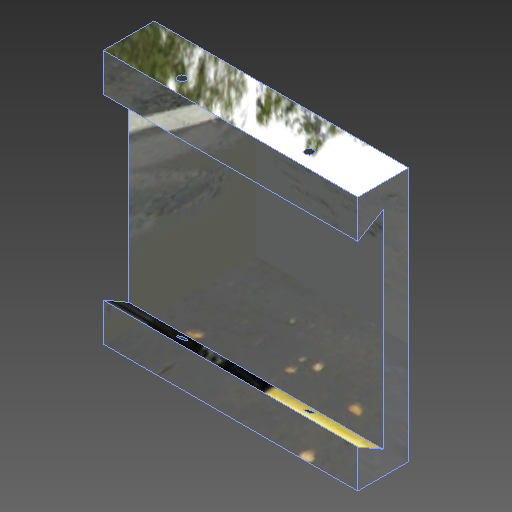
# Autodesk Inventor part: 3d_LM-Welding_Tooling - Fixed base
Saved by Autodesk Inventor 2018.3 (Build 223284000, 284)
## iProperties
Created: 2026-01-13
Part Number: 3d_LM-Welding_Tooling - Fixed base
Material: Aluminium 6061-T6
Document SubType Name: Modeling
Designer: aca6
Density: 2.7 g/cm^3
Appearance: N/A - Machined Aluminium
Manufacturer-1: {"Name": "Hanstar Technologies Co., Ltd", "PartNumber": "3d_Welding_Tooling - Fixed base", "Link": ""}
Manufacturer-2: {"Name": "SHENZHEN JINYIHE PROTOTYPE TECHNOLOGIES CO., LTD", "PartNumber": "3d_Welding_Tooling - Fixed base", "Link": ""}
Manufacturer-3: {"Name": "Shenzhen city Xavier Precision Co., Ltd.", "PartNumber": "3d_Welding_Tooling - Fixed base", "Link": ""}
Manufacturer-4: {"Name": "", "PartNumber": "", "Link": ""}
Manufacturer-5: {"Name": "", "PartNumber": "", "Link": ""}
Provider-1: {"Name": "", "PartNumber": "", "Link": ""}
Provider-2: {"Name": "", "PartNumber": "", "Link": ""}
Provider-3: {"Name": "", "PartNumber": "", "Link": ""}
Provider-4: {"Name": "", "PartNumber": "", "Link": ""}
Provider-5: {"Name": "", "PartNumber": "", "Link": ""}
Author: aca6
Comments: DIN-ISO-2768-fH
Autodesk Inventor part; units mm, degrees
ref_plane "YZ Plane" through (0, 0, 0) normal (1, 0, 0) x (0, 1, 0)
ref_plane "XZ Plane" through (0, 0, 0) normal (0, 1, 0) x (-1, 0, 0)
ref_plane "XY Plane" through (0, 0, 0) normal (0, 0, 1) x (1, 0, 0)
sketch "Sketch1" plane through (0, 0, 0) normal (0, 0, 1) x (1, 0, 0)
  line L0 (-50, 50) -> (50, 50)
  line L1 (50, 50) -> (50, -50)
  line L2 (50, -50) -> (-50, -50)
  line L3 (-50, -50) -> (-50, 50)
  line L4 (0, 0) -> (0, 7.629) construction
  line L5 (0, 0) -> (6.8797, 0) construction
  dimension "d0" = 100
  dimension "d1" = 100
  constraints: 12 end point, 3 horizontal, 2 parallel, 2 vertical, 1 perpendicular, 4 other
  measures "d0" distance between parallel lines of L2 L0
  measures "d1" distance between parallel lines of L1 L3
extrude "Extrusion1" add sketch "Sketch1" along normal blind 20
sketch "Sketch2" plane through (50, -50, 0) normal (1, 0, 0) x (0, 0, -1)
  line L0 (-20, 100) -> (-20, 0) projected
  line L1 (-20, 15) -> (-10, 9.2265)
  line L2 (-10, 9.2265) -> (-10, 90.7735)
  line L3 (-10, 90.7735) -> (-20, 85)
  line L4 (0, 0) -> (-20, 0) projected
  line L5 (0, 100) -> (-20, 100) projected
  point P0 (0, 50)
  dimension "d4" = 60
  dimension "d5" = 60
  dimension "d6" = 10
  dimension "d7" = 15
  dimension "d8" = 15
  constraints: 6 end point, 2 point on line, 1 parallel
  measures "d4" angle of L2 L1
  measures "d5" angle of L2 L3
  measures "d6" distance between parallel lines of L0 L2
  measures "d7" distance from line of L4 L1.start
  measures "d8" distance from line of L5 L3.end
extrude "Extrusion2" cut sketch "Sketch2" against normal blind 118.25
sketch "Sketch3" plane through (-50, -50, 0) normal (0, -1, 0) x (1, 0, 0)
  line L0 (100, 10) -> (0, 10) projected
  line L1 (0, 0) -> (0, 20) projected
  line L2 (0, 20) -> (100, 20) projected
  line L3 (100, 0) -> (100, 20) projected
  point P0 (50, 0)
  point P1 (25, 14)
  point P2 (75, 14)
  dimension "d11" = 25
  dimension "d12" = 6
  dimension "d21" = 25
  constraints: 1 horizontal alignment
  measures "d11" distance from line of L1 point (25, 14)
  measures "d12" distance from line of L2 point (25, 14)
  measures "d21" distance from line of L3 point (75, 14)
hole "Hole1" at (-25, -50, 14) at (25, -50, 14) direction (0, 1, 0) diameter 3.242 end through all thread size "M4x0.7" class "6H" standard "ISO Metric profile"
sketch "Sketch4" plane through (-50, -50, 0) normal (0, -1, 0) x (1, 0, 0)
  circle A0 centre (5, 5) radius 1.6 projected
  circle A1 centre (14, 5) radius 1.6 projected
  point P0 (50, 0)
  constraints: 2 coincident
hole "Hole2" at (-45, -50, 5) at (-36, -50, 5) direction (0, 1, 0) diameter 2.459 depth 9 tip angle 118 thread size "M3x0.5" class "6H" standard "ISO Metric profile"
body "Solid1"
